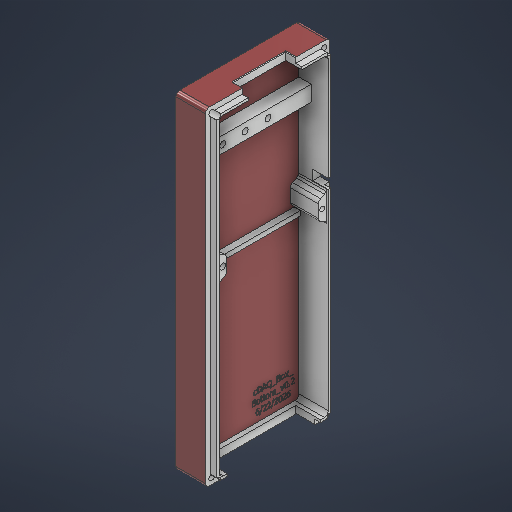
# Autodesk Inventor part: cDAQ_Box_Bottom_v0.2
Saved by Autodesk Inventor 2027 (Build 310192000, 192)
## iProperties
Created: 2026-05-08
Part Number: cDAQ_Box_Bottom_v0.2
Material: Generic
Document SubType Name: Modeling
Designer: giese
Density: 1 g/cm^3
Appearance: Default
Author: giese
Autodesk Inventor part; units mm, degrees
(part 1 of 2)
ref_plane "YZ Plane" through (0, 0, 0) normal (1, 0, 0) x (0, 1, 0)
ref_plane "XZ Plane" through (0, 0, 0) normal (0, 1, 0) x (-1, 0, 0)
ref_plane "XY Plane" through (0, 0, 0) normal (0, 0, 1) x (1, 0, 0)
sketch "Sketch1" plane through (0, 0, 0) normal (1, 0, 0) x (0, 1, 0)
  line L0 (37.5698, 53.1667) -> (-230.1462, 53.1667)
  line L1 (-230.1462, 53.1667) -> (-230.1462, -48.4333)
  line L2 (-230.1462, -48.4333) -> (37.5698, -48.4333)
  line L3 (37.5698, -48.4333) -> (37.5698, 53.1667)
  point P0 (0, 0)
  dimension "d0" = 101.6
  dimension "d1" = 267.716
  constraints: 8 end point, 2 parallel, 1 horizontal, 1 perpendicular
  measures "d0" distance of L2.end L0.start
  measures "d1" distance of L1.end L2.end
extrude "Extrusion1" add sketch "Sketch1" along normal blind 24.13
sketch "Sketch2" plane through (24.13, 0, 0) normal (1, 0, 0) x (0, 0, -1)
  line L0 (42.0833, 31.2198) -> (-46.8167, 31.2198)
  line L1 (-46.8167, 31.2198) -> (-46.8167, -223.7962)
  line L2 (-46.8167, -223.7962) -> (42.0833, -223.7962)
  line L3 (42.0833, -223.7962) -> (42.0833, 31.2198)
  line L4 (48.4333, 37.5698) -> (-53.1667, 37.5698) projected
  line L5 (-53.1667, 37.5698) -> (-53.1667, -230.1462) projected
  line L6 (-53.1667, -230.1462) -> (48.4333, -230.1462) projected
  point P0 (0, 0)
  dimension "d4" = 255.016
  dimension "d5" = 88.9
  dimension "d8" = 6.35
  dimension "d21" = 6.35
  dimension "d690" = 6.35
  constraints: 8 end point, 2 parallel, 1 horizontal, 1 perpendicular
  measures "d4" distance of L2.end L0.start
  measures "d5" distance of L0.start L0.end
  measures "d8" distance between parallel lines of L0 L4
  measures "d21" distance between parallel lines of L5 L1
  measures "d690" distance between parallel lines of L6 L2
extrude "Extrusion2" cut sketch "Sketch2" against normal blind 19.05
sketch "Sketch3" plane through (0, 0, 0) normal (-1, 0, 0) x (0, 0, 1)
  circle A0 centre (-6.6909, -3.0702) radius 2.4005
  circle A1 centre (11.8079, -3.0702) radius 2.4005
  circle A2 centre (30.3067, -3.0702) radius 2.4005
  line L0 (-48.4333, -230.1462) -> (-48.4333, 37.5698) projected
  line L1 (-48.4333, 37.5698) -> (53.1667, 37.5698) projected
  line L2 (53.1667, 37.5698) -> (53.1667, -230.1462) projected
  line L3 (46.8167, 31.2198) -> (-42.0833, 31.2198) projected
  point P0 (0, 0)
  point P1 (-0.896, -23.7433)
  point P2 (-45.1848, 27.0137)
  dimension "d9" = 18.4988
  dimension "d10" = 4.801
  dimension "d11" = 4.801
  dimension "d12" = 18.4988
  dimension "d13" = 36.9976
  dimension "d18" = 22.86
  dimension "d22" = 4.801
  dimension "d58" = 40.64
  constraints: 3 centre point
  measures "d9" distance of A0.centre A1.centre
  measures "d10" diameter of A1
  measures "d11" diameter of A2
  measures "d12" distance of A1.centre A2.centre
  measures "d13" distance of A0.centre A2.centre
  measures "d18" distance from line of L2 A2.centre
  measures "d22" diameter of A0
  measures "d58" distance from line of L1 A2.centre
extrude "Extrusion3" cut sketch "Sketch3" against normal blind 5.08
sketch "Sketch5" plane through (0, -230.1462, -48.4333) normal (0, 0, -1) x (-1, 0, 0)
  line L0 (-27.2034, 165.862) -> (-16.51, 165.862)
  line L1 (-16.51, 165.862) -> (-16.51, 173.862)
  line L2 (-16.51, 173.862) -> (-27.2034, 173.862)
  line L3 (-27.2034, 173.862) -> (-27.2034, 165.862)
  line L4 (0, 267.716) -> (-24.13, 267.716) projected
  line L5 (0, 0) -> (0, 267.716) projected
  line L6 (-24.13, 0) -> (-24.13, 267.716) projected
  point P0 (0, 230.1462)
  point P1 (-21.8567, 173.862)
  point P2 (-21.8567, 165.862)
  dimension "d28" = 10.6934
  dimension "d30" = 8
  dimension "d31" = 16.51
  dimension "d34" = 101.854
  dimension "d215" = 3.0734
  constraints: 8 end point, 2 midpoint, 2 parallel, 1 horizontal, 1 perpendicular
  measures "d28" distance between parallel lines of L1 L3
  measures "d30" distance of point (-21.857, 173.862) point (-21.857, 165.862)
  measures "d31" distance between parallel lines of L5 L1
  measures "d34" distance between parallel lines of L4 L0
  measures "d215" distance between parallel lines of L6 L3
extrude "Extrusion4" cut sketch "Sketch5" against normal blind 24.13
sketch "Sketch6" plane through (0, -230.1462, -48.4333) normal (0, -1, 0) x (1, 0, 0)
  line L0 (24.08, 55.136) -> (16.08, 55.136)
  line L1 (16.08, 45.136) -> (24.08, 45.136)
  line L2 (0, 101.6) -> (0, 0) projected
  line L3 (29.63, 53.1359) -> (29.63, 47.136)
  line L4 (24.08, 55.136) -> (29.63, 53.1359)
  line L5 (29.63, 47.136) -> (24.08, 45.136)
  line L6 (0, 0) -> (24.13, 0) projected
  line L7 (24.13, 95.25) -> (24.13, 6.35) projected
  line L8 (24.13, 41.9134) -> (24.13, 37.4697)
  line L9 (16.08, 55.136) -> (8.636, 55.136)
  line L10 (8.636, 55.136) -> (8.636, 45.136)
  line L11 (8.636, 45.136) -> (21.16, 45.136)
  point P0 (0, 48.4333)
  point P1 (20.08, 55.136)
  point P2 (20.08, 45.136)
  point P3 (16.08, 50.136)
  dimension "d39" = 6
  dimension "d48" = 55.136
  dimension "d221" = 0
  dimension "d223" = 2
  dimension "d224" = 2
  dimension "d225" = 5.5
  dimension "d227" = 5.55
  dimension "d672" = 8.636
  constraints: 18 end point, 2 horizontal, 2 midpoint, 2 parallel, 2 point on line, 1 perpendicular, 1 vertical
  measures "d39" distance of L3.start L3.end
  measures "d48" distance between parallel lines of L6 L0
  measures "d221" horizontal distance of L0.start L1.end
  measures "d223" vertical distance of L3.end L1.end
  measures "d224" vertical distance of L0.start L3.start
  measures "d225" distance between parallel lines of L3 L7
  measures "d227" distance from line of L1.end L3
  measures "d672" distance between parallel lines of L2 L10
extrude "Extrusion5" [suppressed]
sketch "Sketch7" plane through (0, 37.5698, 53.1667) normal (0, 1, 0) x (1, 0, 0)
  line L0 (32.512, 73.66) -> (16.002, 73.66)
  line L1 (16.002, 73.66) -> (16.002, 30.48)
  line L2 (16.002, 30.48) -> (32.512, 30.48)
  line L3 (32.512, 30.48) -> (32.512, 73.66)
  line L4 (0, 0) -> (24.13, 0) projected
  line L5 (0, 101.6) -> (0, 0) projected
  line L6 (24.13, 101.6) -> (24.13, 0) projected
  point P0 (0, 53.1667)
  point P1 (24.13, 73.66)
  point P2 (24.13, 30.48)
  dimension "d51" = 43.18
  dimension "d52" = 30.48
  dimension "d55" = 16.002
  dimension "d56" = 16.51
  dimension "d57" = 8.382
  constraints: 8 end point, 2 parallel, 1 horizontal, 1 perpendicular
  measures "d51" distance of L2.end L0.start
  measures "d52" distance between parallel lines of L4 L2
  measures "d55" distance between parallel lines of L5 L1
  measures "d56" distance between parallel lines of L3 L1
  measures "d57" distance between parallel lines of L6 L3
extrude "Extrusion6" cut sketch "Sketch7" against normal blind 7.62
fillet "Fillet1" radius 3.175 4 edges at (12.065, 37.5698, -48.4333) (12.065, 37.5698, 53.1667) (12.065, -230.1462, -48.4333) (12.065, -230.1462, 53.1667)
sketch "Sketch8" plane through (0, 0, 0) normal (-1, 0, 0) x (0, 0, 1)
  line L0 (-8.4625, -6.6008) -> (-4.9319, -6.6008)
  line L1 (-8.4625, 0.4604) -> (-4.9319, 0.4604)
  line L2 (-8.4625, -6.6008) -> (-10.5009, -3.0702)
  line L3 (-8.4625, 0.4604) -> (-10.5009, -3.0702)
  line L4 (-4.9319, -6.6008) -> (-2.8936, -3.0702)
  line L5 (-4.9319, 0.4604) -> (-2.8936, -3.0702)
  circle A0 centre (-6.6909, -3.0702) radius 2.4005 projected
  line L6 (10.0363, -6.6008) -> (13.5669, -6.6008)
  line L7 (10.0363, 0.4604) -> (13.5669, 0.4604)
  line L8 (10.0363, -6.6008) -> (7.9979, -3.0702)
  line L9 (10.0363, 0.4604) -> (7.9979, -3.0702)
  line L10 (13.5669, -6.6008) -> (15.6053, -3.0702)
  line L11 (13.5669, 0.4604) -> (15.6053, -3.0702)
  circle A1 centre (11.8079, -3.0702) radius 2.4005 projected
  line L12 (28.5351, -6.6008) -> (26.4967, -3.0702)
  line L13 (28.5351, 0.4604) -> (26.4967, -3.0702)
  line L14 (28.5351, -6.6008) -> (32.0657, -6.6008)
  line L15 (28.5351, 0.4604) -> (32.0657, 0.4604)
  line L16 (32.0657, -6.6008) -> (34.1041, -3.0702)
  line L17 (32.0657, 0.4604) -> (34.1041, -3.0702)
  circle A2 centre (30.3067, -3.0702) radius 2.4005 projected
  point P0 (-6.6972, -6.6008)
  point P1 (11.8016, -6.6008)
  point P2 (30.3004, -6.6008)
  point P3 (-10.5009, -3.0702)
  point P4 (-2.8936, -3.0702)
  point P5 (15.6053, -3.0702)
  point P6 (7.9979, -3.0702)
  point P7 (34.1041, -3.0702)
  point P8 (26.4967, -3.0702)
  dimension "d60" = 7.0612
  dimension "d61" = 120
  dimension "d62" = 120
  dimension "d63" = 120
  dimension "d64" = 120
  dimension "d65" = 3.5306
  dimension "d66" = 3.5306
  dimension "d67" = 3.5306
  dimension "d68" = 3.5306
  dimension "d69" = 3.5306
  dimension "d70" = 3.5306
  dimension "d71" = 0
  dimension "d72" = 7.6074
  dimension "d73" = 3.81
  dimension "d74" = 0
  dimension "d75" = 7.0612
  dimension "d76" = 120
  dimension "d77" = 120
  dimension "d78" = 120
  dimension "d79" = 120
  dimension "d80" = 3.5306
  dimension "d81" = 3.5306
  dimension "d82" = 3.5306
  dimension "d83" = 3.5306
  dimension "d84" = 3.5306
  dimension "d85" = 3.5306
  dimension "d86" = 0
  dimension "d87" = 7.6074
  dimension "d91" = 0
  dimension "d92" = 3.81
  dimension "d93" = 7.0612
  dimension "d94" = 120
  dimension "d95" = 120
  dimension "d96" = 120
  dimension "d97" = 120
  dimension "d98" = 3.5306
  dimension "d99" = 3.5306
  dimension "d100" = 3.5306
  dimension "d101" = 3.5306
  dimension "d102" = 3.5306
  dimension "d103" = 3.5306
  dimension "d104" = 0
  dimension "d105" = 7.6074
  dimension "d108" = 0
  dimension "d109" = 3.81
  constraints: 36 end point, 6 horizontal, 3 midpoint
  measures "d60" distance from line of point (-6.697, -6.601) L1
  measures "d61" angle of L0 L2
  measures "d62" angle of L1 L3
  measures "d63" angle of L4 L0
  measures "d64" angle of L5 L1
  measures "d65" distance of L0.start L0.end
  measures "d66" distance of L1.start L1.end
  measures "d67" vertical distance of L1.start L3.end
  measures "d68" vertical distance of L0.start L2.end
  measures "d69" vertical distance of L1.end L5.end
  measures "d70" vertical distance of L0.end L4.end
  measures "d71" horizontal distance of L0.start L1.start
  measures "d72" distance of L4.end L2.end
  measures "d73" distance of A0.centre L2.end
  measures "d74" vertical distance of A0.centre L4.end
  measures "d75" distance from line of point (11.802, -6.601) L7
  measures "d76" angle of L6 L8
  measures "d77" angle of L7 L9
  measures "d78" angle of L10 L6
  measures "d79" angle of L11 L7
  measures "d80" distance of L8.start L6.end
  measures "d81" distance of L9.start L7.end
  measures "d82" vertical distance of L9.start L9.end
  measures "d83" vertical distance of L8.start L8.end
  measures "d84" vertical distance of L7.end L11.end
  measures "d85" vertical distance of L6.end L10.end
  measures "d86" horizontal distance of L8.start L9.start
  measures "d87" distance of L10.end L8.end
  measures "d91" vertical distance of A1.centre L8.end
  measures "d92" distance of A1.centre L8.end
  measures "d93" distance from line of point (30.3, -6.601) L15
  measures "d94" angle of L14 L12
  measures "d95" angle of L15 L13
  measures "d96" angle of L16 L14
  measures "d97" angle of L17 L15
  measures "d98" distance of L12.start L16.start
  measures "d99" distance of L15.start L15.end
  measures "d100" vertical distance of L15.start L13.end
  measures "d101" vertical distance of L12.start L12.end
  measures "d102" vertical distance of L15.end L17.end
  measures "d103" vertical distance of L16.start L16.end
  measures "d104" horizontal distance of L12.start L15.start
  measures "d105" distance of L16.end L12.end
  measures "d108" vertical distance of A2.centre L12.end
  measures "d109" distance of A2.centre L12.end
extrude "Extrusion7" cut sketch "Sketch8" against normal blind 4 contours L2 L3 L1 L5 L4 L0 | A0 | L8 L9 L7 L11 L10 L6 | A1 | L12 L13 L15 L17 L16 L14 | A2
sketch "Sketch9" plane through (5.08, 0, 0) normal (1, 0, 0) x (0, 0, -1)
  arc A0 (24.8089, -180.8044) -> (19.3527, -180.8044) centre (22.0808, -178.3302) ccw
  line L0 (45.2583, 37.5698) -> (20.4933, 37.5698) projected
  line L1 (42.0833, 31.2198) -> (42.0833, -223.7962) projected
  arc A1 (20.1758, -185.9502) -> (23.9858, -185.9502) centre (22.0808, -185.9502) ccw
  line L2 (23.9858, -185.9502) -> (23.9858, -182.9374)
  line L3 (20.1758, -185.9502) -> (20.1758, -182.9374)
  arc A2 (24.8089, -180.8044) -> (23.9858, -182.9374) centre (27.1608, -182.9374) ccw
  arc A3 (20.1758, -182.9374) -> (19.3527, -180.8044) centre (17.0008, -182.9374) ccw
  arc A4 (-25.9911, -180.8044) -> (-31.4473, -180.8045) centre (-28.7192, -178.3302) ccw
  arc A5 (-30.6242, -185.9366) -> (-26.8142, -185.9502) centre (-28.7192, -185.9502) ccw
  line L4 (-26.8142, -185.9502) -> (-26.8142, -182.9374)
  line L5 (-30.6242, -185.9366) -> (-30.6242, -182.9374)
  arc A6 (-25.9911, -180.8044) -> (-26.8142, -182.9374) centre (-23.6392, -182.9374) ccw
  arc A7 (-30.6242, -182.9374) -> (-31.4473, -180.8045) centre (-33.7992, -182.9374) ccw
  line L6 (-22.6867, 37.5698) -> (-49.9917, 37.5698) projected
  line L7 (-46.8167, -223.7962) -> (-46.8167, 31.2198) projected
  point P0 (0, 0)
  point P1 (23.9858, -181.4823)
  point P2 (20.1758, -181.4823)
  point P3 (-26.8142, -181.4823)
  point P4 (-30.6242, -181.4823)
  dimension "d112" = 215.9
  dimension "d114" = 7.366
  dimension "d116" = 3.81
  dimension "d117" = 223.52
  dimension "d118" = 3.175
  dimension "d119" = 7.366
  dimension "d120" = 3.81
  dimension "d121" = 3.175
  dimension "d122" = 215.9
  dimension "d123" = 223.52
  dimension "d125" = 0
  dimension "d128" = 50.8
  dimension "d129" = 20.0025
  dimension "d130" = 0
  constraints: 20 point on circle, 8 centre point, 8 end point, 8 tangent, 4 point on line, 2 equal radius, 2 parallel, 2 vertical
  measures "d112" distance from line of L0 A0.centre
  measures "d114" diameter of A0
  measures "d116" diameter of A1
  measures "d117" distance from line of L0 A1.centre
  measures "d118" radius of A2
  measures "d119" diameter of A4
  measures "d120" diameter of A5
  measures "d121" radius of A6
  measures "d122" distance from line of A4.centre L6
  measures "d123" distance from line of L6 A5.centre
  measures "d125" horizontal distance of A5.centre A4.centre
  measures "d128" distance of A5.centre A1.centre
  measures "d129" distance from line of L1 A0.centre
  measures "d130" horizontal distance of A0.centre A1.centre
extrude "Extrusion8" [suppressed]
sketch "Sketch10" plane through (24.13, 0, 0) normal (1, 0, 0) x (0, 0, -1)
  line L0 (-46.8167, 31.2198) -> (42.0833, 31.2198) projected
  line L1 (-46.8167, 31.2198) -> (42.0833, 31.2198)
  line L2 (42.0833, 33.2264) -> (-46.8167, 33.2264)
  line L3 (-46.8167, 33.2264) -> (-48.8233, 33.2264)
  line L4 (-48.8233, 33.2264) -> (-48.8233, -225.8028)
  line L5 (-48.8233, -225.8028) -> (44.0899, -225.8028)
  line L6 (44.0899, -225.8028) -> (44.0899, 33.2264)
  line L7 (44.0899, 33.2264) -> (41.9392, 33.2264)
  line L8 (42.0833, 31.2198) -> (42.0833, -223.7962) projected
  line L9 (-46.8167, -223.7962) -> (-46.8167, 31.2198) projected
  line L10 (42.0833, -223.7962) -> (-46.8167, -223.7962) projected
  line L11 (45.2583, 37.5698) -> (20.4933, 37.5698) projected
  dimension "d202" = 2.0066
  dimension "d203" = 2.0066
  dimension "d204" = 2.0066
  dimension "d205" = 2.0066
  dimension "d208" = 4.3434
  constraints: 14 end point, 3 perpendicular, 3 point on line, 1 collinear, 1 horizontal
  measures "d202" distance between parallel lines of L0 L2
  measures "d203" distance between parallel lines of L6 L8
  measures "d204" distance between parallel lines of L4 L9
  measures "d205" distance between parallel lines of L5 L10
  measures "d208" distance between parallel lines of L11 L2
extrude "Extrusion9" add sketch "Sketch10" along normal blind 5
fillet "Fillet2" radius 3.175 8 edges at (17.105, 31.2198, -42.0833) (17.105, 31.2198, 46.8167) (17.105, -223.7962, 46.8167) (17.105, -223.7962, -42.0833) (26.63, 33.2264, -44.0899) (26.63, 33.2264, 48.8233) (26.63, -225.8028, -44.0899) (26.63, -225.8028, 48.8233)
sketch "Sketch13" plane through (29.13, 0, 0) normal (1, 0, 0) x (0, 0, -1)
  arc A0 (44.0833, 30.0448) -> (40.9083, 33.2198) centre (40.9083, 30.0448) ccw projected
  arc A1 (-45.6417, 33.2198) -> (-48.8167, 30.0448) centre (-45.6417, 30.0448) ccw projected
  arc A2 (40.9083, -212.0802) -> (44.0833, -208.9052) centre (40.9083, -208.9052) ccw projected
  arc A3 (-48.8167, -208.9052) -> (-45.6417, -212.0802) centre (-45.6417, -208.9052) ccw projected
  line L0 (-22.6867, 37.5698) -> (-49.9917, 37.5698) projected
  line L1 (-53.1667, 34.3948) -> (-53.1667, -226.9712) projected
  line L2 (-49.9917, -230.1462) -> (45.2583, -230.1462) projected
  arc A4 (-48.8167, -208.9052) -> (-45.6417, -212.0802) centre (-45.6417, -208.9052) ccw projected
  circle A5 centre (-48.0867, -225.0662) radius 2.4005
  circle A6 centre (43.3533, -225.0662) radius 2.4005
  line L3 (48.4333, -226.9712) -> (48.4333, 34.3948) projected
  circle A7 centre (43.3533, 32.4898) radius 2.4005
  line L4 (45.2583, 37.5698) -> (20.4933, 37.5698) projected
  circle A8 centre (-48.0867, 32.4898) radius 2.4005
  arc A9 (41.4904, -28.6131) -> (38.3154, -25.4381) centre (38.3154, -28.6131) ccw
  circle A10 centre (38.2733, -76.7302) radius 2.4005
  circle A11 centre (-43.0067, -76.7302) radius 2.4005
  point P0 (0, 0)
  point P1 (-47.8868, 32.2898)
  point P2 (-47.8868, -211.1503)
  point P3 (-47.8868, -211.1503)
  point P4 (45.8404, -24.2631)
  point P5 (42.6654, -21.0881)
  dimension "d178" = 5.08
  dimension "d179" = 5.08
  dimension "d180" = 4.801
  dimension "d181" = 5.08
  dimension "d182" = 5.08
  dimension "d183" = 4.801
  dimension "d184" = 4.801
  dimension "d185" = 5.08
  dimension "d186" = 5.08
  dimension "d187" = 4.801
  dimension "d188" = 5.08
  dimension "d189" = 5.08
  dimension "d326" = 4.801
  dimension "d327" = 10.16
  dimension "d328" = 114.3
  dimension "d329" = 4.801
  dimension "d330" = 10.16
  dimension "d331" = 114.3
  constraints: 7 centre point, 5 point on circle
  measures "d178" distance from line of L1 A5.centre
  measures "d179" distance from line of L2 A5.centre
  measures "d180" diameter of A5
  measures "d181" distance from line of L2 A6.centre
  measures "d182" distance from line of L3 A6.centre
  measures "d183" diameter of A6
  measures "d184" diameter of A7
  measures "d185" distance from line of L3 A7.centre
  measures "d186" distance from line of L4 A7.centre
  measures "d187" diameter of A8
  measures "d188" distance from line of L0 A8.centre
  measures "d189" distance from line of L1 A8.centre
  measures "d326" diameter of A10
  measures "d327" distance from line of L3 A10.centre
  measures "d328" distance from line of A10.centre L4
  measures "d329" diameter of A11
  measures "d330" distance from line of L1 A11.centre
  measures "d331" distance from line of L0 A11.centre
extrude "Extrusion11" cut sketch "Sketch13" against normal blind 25.4
sketch "Sketch14" plane through (5.08, 0, 0) normal (1, 0, 0) x (0, 0, -1)
  line L0 (11.5819, -199.2242) -> (30.7986, -199.2242) construction
  line L1 (30.7986, -199.2242) -> (30.7986, -197.2748) construction
  line L2 (30.7986, -197.2748) -> (11.5819, -197.2748) construction
  line L3 (11.5819, -197.2748) -> (11.5819, -199.2242) construction
  spline S0 degree 2 poles (6.6851, -203.9704) (6.3294, -203.9704) (5.7403, -203.7518) (5.5291, -203.5295) knots 0 0 0 1 2 2 2
  spline S1 degree 2 poles (5.5291, -203.5295) (5.3179, -203.3109) (5.0845, -202.6366) (5.0845, -202.1846) knots 0 0 0 1 2 2 2
  spline S2 degree 2 poles (5.0845, -202.1846) (5.0845, -201.7325) (5.3253, -201.073) (5.5291, -200.8507) knots 0 0 0 1 2 2 2
  spline S3 degree 2 poles (5.5291, -200.8507) (5.7329, -200.6247) (6.3368, -200.3839) (6.6851, -200.3839) knots 0 0 0 1 2 2 2
  spline S4 degree 2 poles (6.6851, -200.3839) (6.9667, -200.3839) (7.4928, -200.5432) (7.6966, -200.647) knots 0 0 0 1 2 2 2
  line L4 (7.6966, -200.647) -> (7.6966, -201.2953)
  line L5 (7.6966, -201.2953) -> (7.6632, -201.2953)
  spline S5 degree 2 poles (7.6632, -201.2953) (7.6002, -201.2435) (7.4076, -201.1101) (7.2705, -201.0397) knots 0 0 0 1 2 2 2
  spline S6 degree 2 poles (7.2705, -201.0397) (7.1482, -200.9804) (6.8222, -200.8878) (6.674, -200.8878) knots 0 0 0 1 2 2 2
  spline S7 degree 2 poles (6.674, -200.8878) (6.2257, -200.8878) (5.681, -201.5658) (5.681, -202.1846) knots 0 0 0 1 2 2 2
  spline S8 degree 2 poles (5.681, -202.1846) (5.681, -202.7885) (6.2071, -203.4665) (6.674, -203.4665) knots 0 0 0 1 2 2 2
  spline S9 degree 2 poles (6.674, -203.4665) (6.9556, -203.4665) (7.4668, -203.2331) (7.6632, -203.0515) knots 0 0 0 1 2 2 2
  line L6 (7.6632, -203.0515) -> (7.6966, -203.0515)
  line L7 (7.6966, -203.0515) -> (7.6966, -203.6999)
  spline S10 degree 2 poles (7.6966, -203.6999) (7.6113, -203.7407) (7.352, -203.8555) (7.2483, -203.8815) knots 0 0 0 1 2 2 2
  spline S11 degree 2 poles (7.2483, -203.8815) (7.1, -203.9259) (6.8666, -203.9704) (6.6851, -203.9704) knots 0 0 0 1 2 2 2
  spline S12 degree 2 poles (11.8721, -201.6103) (11.8721, -202.2364) (11.3645, -203.2442) (10.9385, -203.5258) knots 0 0 0 1 2 2 2
  spline S13 degree 2 poles (10.9385, -203.5258) (10.5902, -203.7444) (9.8751, -203.8926) (9.3194, -203.8926) knots 0 0 0 1 2 2 2
  line L8 (9.3194, -203.8926) -> (8.2671, -203.8926)
  line L9 (8.2671, -203.8926) -> (8.2671, -199.3206)
  line L10 (8.2671, -199.3206) -> (9.3082, -199.3206)
  spline S14 degree 2 poles (9.3082, -199.3206) (9.9529, -199.3206) (10.6865, -199.5132) (10.9459, -199.6837) knots 0 0 0 1 2 2 2
  spline S15 degree 2 poles (10.9459, -199.6837) (11.3868, -199.9764) (11.8721, -200.9434) (11.8721, -201.6103) knots 0 0 0 1 2 2 2
  spline S16 degree 2 poles (11.2386, -201.6029) (11.2386, -201.0767) (10.8903, -200.332) (10.5457, -200.1209) knots 0 0 0 1 2 2 2
  spline S17 degree 2 poles (10.5457, -200.1209) (10.3012, -199.9764) (9.7491, -199.8467) (9.3379, -199.8467) knots 0 0 0 1 2 2 2
  line L11 (9.3379, -199.8467) -> (8.8748, -199.8467)
  line L12 (8.8748, -199.8467) -> (8.8748, -203.3665)
  line L13 (8.8748, -203.3665) -> (9.3379, -203.3665)
  spline S18 degree 2 poles (9.3379, -203.3665) (9.7417, -203.3665) (10.3531, -203.2368) (10.6013, -203.0626) knots 0 0 0 1 2 2 2
  spline S19 degree 2 poles (10.6013, -203.0626) (10.9199, -202.8478) (11.2386, -202.1364) (11.2386, -201.6029) knots 0 0 0 1 2 2 2
  line L14 (12.0388, -203.8926) -> (13.5801, -199.3206)
  line L15 (13.5801, -199.3206) -> (14.3286, -199.3206)
  line L16 (14.3286, -199.3206) -> (15.8698, -203.8926)
  line L17 (15.8698, -203.8926) -> (15.2289, -203.8926)
  line L18 (15.2289, -203.8926) -> (14.8139, -202.6143)
  line L19 (14.8139, -202.6143) -> (13.0688, -202.6143)
  line L20 (13.0688, -202.6143) -> (12.6539, -203.8926)
  line L21 (12.6539, -203.8926) -> (12.0388, -203.8926)
  line L22 (14.6472, -202.0956) -> (13.9395, -199.943)
  line L23 (13.9395, -199.943) -> (13.2356, -202.0956)
  line L24 (13.2356, -202.0956) -> (14.6472, -202.0956)
  spline S20 degree 2 poles (20.101, -205.0115) (19.9343, -205.0522) (19.5712, -205.0967) (19.3896, -205.0967) knots 0 0 0 1 2 2 2
  spline S21 degree 2 poles (19.3896, -205.0967) (18.8746, -205.0967) (18.2336, -204.5224) (18.204, -203.9889) knots 0 0 0 1 2 2 2
  spline S22 degree 2 poles (18.204, -203.9889) (18.1633, -203.9889) (18.0929, -203.9889) (18.0632, -203.9889) knots 0 0 0 1 2 2 2
  spline S23 degree 2 poles (18.0632, -203.9889) (17.6001, -203.9889) (16.8554, -203.674) (16.5886, -203.3665) knots 0 0 0 1 2 2 2
  spline S24 degree 2 poles (16.5886, -203.3665) (16.3256, -203.0626) (16.044, -202.1734) (16.044, -201.6103) knots 0 0 0 1 2 2 2
  spline S25 degree 2 poles (16.044, -201.6103) (16.044, -201.0323) (16.3293, -200.1579) (16.5923, -199.8467) knots 0 0 0 1 2 2 2
  spline S26 degree 2 poles (16.5923, -199.8467) (16.8591, -199.5392) (17.6038, -199.2242) (18.0632, -199.2242) knots 0 0 0 1 2 2 2
  spline S27 degree 2 poles (18.0632, -199.2242) (18.53, -199.2242) (19.2785, -199.5503) (19.5378, -199.8467) knots 0 0 0 1 2 2 2
  spline S28 degree 2 poles (19.5378, -199.8467) (19.7972, -200.1468) (20.0862, -201.0397) (20.0862, -201.6103) knots 0 0 0 1 2 2 2
  spline S29 degree 2 poles (20.0862, -201.6103) (20.0862, -202.4995) (19.3933, -203.6554) (18.7894, -203.8592) knots 0 0 0 1 2 2 2
  spline S30 degree 2 poles (18.7894, -203.8592) (18.8042, -204.0297) (18.8931, -204.3038) (18.9635, -204.3816) knots 0 0 0 1 2 2 2
  spline S31 degree 2 poles (18.9635, -204.3816) (19.0488, -204.478) (19.2822, -204.5669) (19.4897, -204.5669) knots 0 0 0 1 2 2 2
  spline S32 degree 2 poles (19.4897, -204.5669) (19.6119, -204.5669) (19.9454, -204.4891) (20.0195, -204.4594) knots 0 0 0 1 2 2 2
  line L25 (20.0195, -204.4594) -> (20.101, -204.4594)
  line L26 (20.101, -204.4594) -> (20.101, -205.0115)
  spline S33 degree 2 poles (19.4526, -201.6103) (19.4526, -201.1546) (19.2562, -200.4543) (19.0784, -200.2246) knots 0 0 0 1 2 2 2
  spline S34 degree 2 poles (19.0784, -200.2246) (18.8968, -199.9875) (18.3856, -199.7504) (18.0669, -199.7504) knots 0 0 0 1 2 2 2
  spline S35 degree 2 poles (18.0669, -199.7504) (17.7372, -199.7504) (17.2407, -199.9801) (17.0517, -200.2246) knots 0 0 0 1 2 2 2
  spline S36 degree 2 poles (17.0517, -200.2246) (16.8702, -200.458) (16.6775, -201.1657) (16.6775, -201.6103) knots 0 0 0 1 2 2 2
  spline S37 degree 2 poles (16.6775, -201.6103) (16.6775, -202.5106) (17.4334, -203.4702) (18.0669, -203.4702) knots 0 0 0 1 2 2 2
  spline S38 degree 2 poles (18.0669, -203.4702) (18.7005, -203.4702) (19.4526, -202.5106) (19.4526, -201.6103) knots 0 0 0 1 2 2 2
  line L27 (23.769, -204.8114) -> (20.2418, -204.8114)
  line L28 (20.2418, -204.8114) -> (20.2418, -204.415)
  line L29 (20.2418, -204.415) -> (23.769, -204.415)
  line L30 (23.769, -204.415) -> (23.769, -204.8114)
  spline S39 degree 2 poles (27.285, -202.4884) (27.285, -202.8292) (27.0257, -203.3516) (26.8108, -203.5221) knots 0 0 0 1 2 2 2
  spline S40 degree 2 poles (26.8108, -203.5221) (26.5514, -203.7221) (25.9623, -203.8926) (25.4955, -203.8926) knots 0 0 0 1 2 2 2
  line L31 (25.4955, -203.8926) -> (24.1839, -203.8926)
  line L32 (24.1839, -203.8926) -> (24.1839, -199.3206)
  line L33 (24.1839, -199.3206) -> (25.3955, -199.3206)
  spline S41 degree 2 poles (25.3955, -199.3206) (25.8845, -199.3206) (26.3736, -199.3836) (26.5959, -199.5058) knots 0 0 0 1 2 2 2
  spline S42 degree 2 poles (26.5959, -199.5058) (26.8441, -199.6355) (27.0701, -200.0616) (27.0701, -200.3506) knots 0 0 0 1 2 2 2
  spline S43 degree 2 poles (27.0701, -200.3506) (27.0701, -200.6729) (26.7293, -201.1842) (26.4292, -201.3287) knots 0 0 0 1 2 2 2
  line L34 (26.4292, -201.3287) -> (26.4292, -201.3509)
  spline S44 degree 2 poles (26.4292, -201.3509) (26.8367, -201.4621) (27.285, -202.0512) (27.285, -202.4884) knots 0 0 0 1 2 2 2
  spline S45 degree 2 poles (26.6515, -202.5143) (26.6515, -202.2549) (26.5033, -201.9215) (26.281, -201.8029) knots 0 0 0 1 2 2 2
  spline S46 degree 2 poles (26.281, -201.8029) (26.1365, -201.7288) (25.7956, -201.6844) (25.4807, -201.6844) knots 0 0 0 1 2 2 2
  line L35 (25.4807, -201.6844) -> (24.7915, -201.6844)
  line L36 (24.7915, -201.6844) -> (24.7915, -203.3739)
  line L37 (24.7915, -203.3739) -> (25.2843, -203.3739)
  spline S47 degree 2 poles (25.2843, -203.3739) (25.6845, -203.3739) (26.1439, -203.2998) (26.3217, -203.1812) knots 0 0 0 1 2 2 2
  spline S48 degree 2 poles (26.3217, -203.1812) (26.4921, -203.0589) (26.6515, -202.7551) (26.6515, -202.5143) knots 0 0 0 1 2 2 2
  spline S49 degree 2 poles (26.4366, -200.4358) (26.4366, -200.2728) (26.3254, -200.0282) (26.2032, -199.9578) knots 0 0 0 1 2 2 2
  spline S50 degree 2 poles (26.2032, -199.9578) (26.055, -199.8763) (25.6956, -199.8393) (25.3732, -199.8393) knots 0 0 0 1 2 2 2
  line L38 (25.3732, -199.8393) -> (24.7915, -199.8393)
  line L39 (24.7915, -199.8393) -> (24.7915, -201.1768)
  line L40 (24.7915, -201.1768) -> (25.4807, -201.1768)
  spline S51 degree 2 poles (25.4807, -201.1768) (25.766, -201.1768) (26.0364, -201.1175) (26.1809, -201.0249) knots 0 0 0 1 2 2 2
  spline S52 degree 2 poles (26.1809, -201.0249) (26.3217, -200.936) (26.4366, -200.6507) (26.4366, -200.4358) knots 0 0 0 1 2 2 2
  spline S53 degree 2 poles (30.664, -202.1771) (30.664, -203.0441) (29.8304, -203.9889) (29.1338, -203.9889) knots 0 0 0 1 2 2 2
  spline S54 degree 2 poles (29.1338, -203.9889) (28.4188, -203.9889) (27.5999, -203.0145) (27.5999, -202.1771) knots 0 0 0 1 2 2 2
  spline S55 degree 2 poles (27.5999, -202.1771) (27.5999, -201.3176) (28.4447, -200.3654) (29.1338, -200.3654) knots 0 0 0 1 2 2 2
  spline S56 degree 2 poles (29.1338, -200.3654) (29.8304, -200.3654) (30.664, -201.3139) (30.664, -202.1771) knots 0 0 0 1 2 2 2
  spline S57 degree 2 poles (30.0675, -202.1771) (30.0675, -201.5102) (29.5821, -200.8619) (29.1338, -200.8619) knots 0 0 0 1 2 2 2
  spline S58 degree 2 poles (29.1338, -200.8619) (28.6855, -200.8619) (28.1965, -201.5102) (28.1965, -202.1771) knots 0 0 0 1 2 2 2
  spline S59 degree 2 poles (28.1965, -202.1771) (28.1965, -202.8255) (28.6855, -203.4924) (29.1338, -203.4924) knots 0 0 0 1 2 2 2
  spline S60 degree 2 poles (29.1338, -203.4924) (29.5784, -203.4924) (30.0675, -202.8366) (30.0675, -202.1771) knots 0 0 0 1 2 2 2
  line L41 (33.9207, -203.8926) -> (33.2131, -203.8926)
  line L42 (33.2131, -203.8926) -> (32.3794, -202.6032)
  line L43 (32.3794, -202.6032) -> (31.5236, -203.8926)
  line L44 (31.5236, -203.8926) -> (30.8678, -203.8926)
  line L45 (30.8678, -203.8926) -> (32.0571, -202.192)
  line L46 (32.0571, -202.192) -> (30.8789, -200.4617)
  line L47 (30.8789, -200.4617) -> (31.5866, -200.4617)
  line L48 (31.5866, -200.4617) -> (32.4165, -201.7399)
  line L49 (32.4165, -201.7399) -> (33.2649, -200.4617)
  line L50 (33.2649, -200.4617) -> (33.9207, -200.4617)
  line L51 (33.9207, -200.4617) -> (32.7388, -202.1549)
  line L52 (32.7388, -202.1549) -> (33.9207, -203.8926)
  line L53 (37.4294, -204.8114) -> (33.9022, -204.8114)
  line L54 (33.9022, -204.8114) -> (33.9022, -204.415)
  line L55 (33.9022, -204.415) -> (37.4294, -204.415)
  line L56 (37.4294, -204.415) -> (37.4294, -204.8114)
  spline S61 degree 2 poles (7.0815, -210.016) (7.0815, -210.3569) (6.8222, -210.8793) (6.6073, -211.0497) knots 0 0 0 1 2 2 2
  spline S62 degree 2 poles (6.6073, -211.0497) (6.3479, -211.2498) (5.7588, -211.4202) (5.292, -211.4202) knots 0 0 0 1 2 2 2
  line L57 (5.292, -211.4202) -> (3.9804, -211.4202)
  line L58 (3.9804, -211.4202) -> (3.9804, -206.8482)
  line L59 (3.9804, -206.8482) -> (5.192, -206.8482)
  spline S63 degree 2 poles (5.192, -206.8482) (5.681, -206.8482) (6.1701, -206.9112) (6.3924, -207.0335) knots 0 0 0 1 2 2 2
  spline S64 degree 2 poles (6.3924, -207.0335) (6.6406, -207.1632) (6.8666, -207.5892) (6.8666, -207.8782) knots 0 0 0 1 2 2 2
  spline S65 degree 2 poles (6.8666, -207.8782) (6.8666, -208.2006) (6.5258, -208.7119) (6.2257, -208.8564) knots 0 0 0 1 2 2 2
  line L60 (6.2257, -208.8564) -> (6.2257, -208.8786)
  spline S66 degree 2 poles (6.2257, -208.8786) (6.6332, -208.9897) (7.0815, -209.5788) (7.0815, -210.016) knots 0 0 0 1 2 2 2
  spline S67 degree 2 poles (6.448, -210.042) (6.448, -209.7826) (6.2998, -209.4492) (6.0775, -209.3306) knots 0 0 0 1 2 2 2
  spline S68 degree 2 poles (6.0775, -209.3306) (5.933, -209.2565) (5.5921, -209.2121) (5.2772, -209.2121) knots 0 0 0 1 2 2 2
  line L61 (5.2772, -209.2121) -> (4.588, -209.2121)
  line L62 (4.588, -209.2121) -> (4.588, -210.9015)
  line L63 (4.588, -210.9015) -> (5.0808, -210.9015)
  spline S69 degree 2 poles (5.0808, -210.9015) (5.481, -210.9015) (5.9404, -210.8274) (6.1182, -210.7089) knots 0 0 0 1 2 2 2
  spline S70 degree 2 poles (6.1182, -210.7089) (6.2886, -210.5866) (6.448, -210.2828) (6.448, -210.042) knots 0 0 0 1 2 2 2
  spline S71 degree 2 poles (6.2331, -207.9635) (6.2331, -207.8004) (6.1219, -207.5559) (5.9997, -207.4855) knots 0 0 0 1 2 2 2
  spline S72 degree 2 poles (5.9997, -207.4855) (5.8515, -207.404) (5.4921, -207.3669) (5.1697, -207.3669) knots 0 0 0 1 2 2 2
  line L64 (5.1697, -207.3669) -> (4.588, -207.3669)
  line L65 (4.588, -207.3669) -> (4.588, -208.7045)
  line L66 (4.588, -208.7045) -> (5.2772, -208.7045)
  spline S73 degree 2 poles (5.2772, -208.7045) (5.5625, -208.7045) (5.8329, -208.6452) (5.9774, -208.5526) knots 0 0 0 1 2 2 2
  spline S74 degree 2 poles (5.9774, -208.5526) (6.1182, -208.4636) (6.2331, -208.1783) (6.2331, -207.9635) knots 0 0 0 1 2 2 2
  spline S75 degree 2 poles (10.4605, -209.7048) (10.4605, -210.5718) (9.6269, -211.5166) (8.9303, -211.5166) knots 0 0 0 1 2 2 2
  spline S76 degree 2 poles (8.9303, -211.5166) (8.2153, -211.5166) (7.3965, -210.5422) (7.3965, -209.7048) knots 0 0 0 1 2 2 2
  spline S77 degree 2 poles (7.3965, -209.7048) (7.3965, -208.8453) (8.2412, -207.8931) (8.9303, -207.8931) knots 0 0 0 1 2 2 2
  spline S78 degree 2 poles (8.9303, -207.8931) (9.6269, -207.8931) (10.4605, -208.8415) (10.4605, -209.7048) knots 0 0 0 1 2 2 2
  spline S79 degree 2 poles (9.864, -209.7048) (9.864, -209.0379) (9.3786, -208.3895) (8.9303, -208.3895) knots 0 0 0 1 2 2 2
  spline S80 degree 2 poles (8.9303, -208.3895) (8.482, -208.3895) (7.993, -209.0379) (7.993, -209.7048) knots 0 0 0 1 2 2 2
  spline S81 degree 2 poles (7.993, -209.7048) (7.993, -210.3532) (8.482, -211.0201) (8.9303, -211.0201) knots 0 0 0 1 2 2 2
  spline S82 degree 2 poles (8.9303, -211.0201) (9.3749, -211.0201) (9.864, -210.3643) (9.864, -209.7048) knots 0 0 0 1 2 2 2
  spline S83 degree 2 poles (12.0907, -211.4869) (11.6202, -211.4869) (11.0904, -210.9497) (11.0904, -210.368) knots 0 0 0 1 2 2 2
  line L67 (11.0904, -210.368) -> (11.0904, -208.4673)
  line L68 (11.0904, -208.4673) -> (10.7013, -208.4673)
  line L69 (10.7013, -208.4673) -> (10.7013, -207.9894)
  line L70 (10.7013, -207.9894) -> (11.0904, -207.9894)
  line L71 (11.0904, -207.9894) -> (11.0904, -207.0039)
  line L72 (11.0904, -207.0039) -> (11.6683, -207.0039)
  line L73 (11.6683, -207.0039) -> (11.6683, -207.9894)
  line L74 (11.6683, -207.9894) -> (12.7317, -207.9894)
  line L75 (12.7317, -207.9894) -> (12.7317, -208.4673)
  line L76 (12.7317, -208.4673) -> (11.6683, -208.4673)
  line L77 (11.6683, -208.4673) -> (11.6683, -210.1013)
  spline S84 degree 2 poles (11.6683, -210.1013) (11.6683, -210.3606) (11.6869, -210.6459) (11.7499, -210.7682) knots 0 0 0 1 2 2 2
  spline S85 degree 2 poles (11.7499, -210.7682) (11.8017, -210.8756) (12.0351, -210.9831) (12.2352, -210.9831) knots 0 0 0 1 2 2 2
  spline S86 degree 2 poles (12.2352, -210.9831) (12.376, -210.9831) (12.6391, -210.8978) (12.6983, -210.8719) knots 0 0 0 1 2 2 2
  line L78 (12.6983, -210.8719) -> (12.7317, -210.8719)
  line L79 (12.7317, -210.8719) -> (12.7317, -211.3906)
  spline S87 degree 2 poles (12.7317, -211.3906) (12.5687, -211.4351) (12.2352, -211.4869) (12.0907, -211.4869) knots 0 0 0 1 2 2 2
  spline S88 degree 2 poles (14.1952, -211.4869) (13.7246, -211.4869) (13.1948, -210.9497) (13.1948, -210.368) knots 0 0 0 1 2 2 2
  line L80 (13.1948, -210.368) -> (13.1948, -208.4673)
  line L81 (13.1948, -208.4673) -> (12.8058, -208.4673)
  line L82 (12.8058, -208.4673) -> (12.8058, -207.9894)
  line L83 (12.8058, -207.9894) -> (13.1948, -207.9894)
  line L84 (13.1948, -207.9894) -> (13.1948, -207.0039)
  line L85 (13.1948, -207.0039) -> (13.7728, -207.0039)
  line L86 (13.7728, -207.0039) -> (13.7728, -207.9894)
  line L87 (13.7728, -207.9894) -> (14.8361, -207.9894)
  line L88 (14.8361, -207.9894) -> (14.8361, -208.4673)
  line L89 (14.8361, -208.4673) -> (13.7728, -208.4673)
  line L90 (13.7728, -208.4673) -> (13.7728, -210.1013)
  spline S89 degree 2 poles (13.7728, -210.1013) (13.7728, -210.3606) (13.7913, -210.6459) (13.8543, -210.7682) knots 0 0 0 1 2 2 2
  spline S90 degree 2 poles (13.8543, -210.7682) (13.9062, -210.8756) (14.1396, -210.9831) (14.3397, -210.9831) knots 0 0 0 1 2 2 2
  spline S91 degree 2 poles (14.3397, -210.9831) (14.4805, -210.9831) (14.7435, -210.8978) (14.8028, -210.8719) knots 0 0 0 1 2 2 2
  line L91 (14.8028, -210.8719) -> (14.8361, -210.8719)
  line L92 (14.8361, -210.8719) -> (14.8361, -211.3906)
  spline S92 degree 2 poles (14.8361, -211.3906) (14.6731, -211.4351) (14.3397, -211.4869) (14.1952, -211.4869) knots 0 0 0 1 2 2 2
  spline S93 degree 2 poles (18.0817, -209.7048) (18.0817, -210.5718) (17.2481, -211.5166) (16.5516, -211.5166) knots 0 0 0 1 2 2 2
  spline S94 degree 2 poles (16.5516, -211.5166) (15.8365, -211.5166) (15.0177, -210.5422) (15.0177, -209.7048) knots 0 0 0 1 2 2 2
  spline S95 degree 2 poles (15.0177, -209.7048) (15.0177, -208.8453) (15.8624, -207.8931) (16.5516, -207.8931) knots 0 0 0 1 2 2 2
  spline S96 degree 2 poles (16.5516, -207.8931) (17.2481, -207.8931) (18.0817, -208.8415) (18.0817, -209.7048) knots 0 0 0 1 2 2 2
  spline S97 degree 2 poles (17.4852, -209.7048) (17.4852, -209.0379) (16.9999, -208.3895) (16.5516, -208.3895) knots 0 0 0 1 2 2 2
  spline S98 degree 2 poles (16.5516, -208.3895) (16.1033, -208.3895) (15.6142, -209.0379) (15.6142, -209.7048) knots 0 0 0 1 2 2 2
  spline S99 degree 2 poles (15.6142, -209.7048) (15.6142, -210.3532) (16.1033, -211.0201) (16.5516, -211.0201) knots 0 0 0 1 2 2 2
  spline S100 degree 2 poles (16.5516, -211.0201) (16.9962, -211.0201) (17.4852, -210.3643) (17.4852, -209.7048) knots 0 0 0 1 2 2 2
  line L93 (22.5648, -211.4202) -> (22.5648, -209.4344)
  spline S101 degree 2 poles (22.5648, -209.4344) (22.5648, -209.1972) (22.5278, -208.7934) (22.4685, -208.6822) knots 0 0 0 1 2 2 2
  spline S102 degree 2 poles (22.4685, -208.6822) (22.4092, -208.56) (22.1832, -208.4414) (21.9868, -208.4414) knots 0 0 0 1 2 2 2
  spline S103 degree 2 poles (21.9868, -208.4414) (21.809, -208.4414) (21.4014, -208.66) (21.1866, -208.8675) knots 0 0 0 1 2 2 2
  spline S104 degree 2 poles (21.1866, -208.8675) (21.1903, -208.9194) (21.1977, -209.0638) (21.1977, -209.1602) knots 0 0 0 1 2 2 2
  line L94 (21.1977, -209.1602) -> (21.1977, -211.4202)
  line L95 (21.1977, -211.4202) -> (20.6197, -211.4202)
  line L96 (20.6197, -211.4202) -> (20.6197, -209.4344)
  spline S105 degree 2 poles (20.6197, -209.4344) (20.6197, -209.1972) (20.5826, -208.7934) (20.5234, -208.6822) knots 0 0 0 1 2 2 2
  spline S106 degree 2 poles (20.5234, -208.6822) (20.4641, -208.56) (20.2381, -208.4414) (20.0417, -208.4414) knots 0 0 0 1 2 2 2
  spline S107 degree 2 poles (20.0417, -208.4414) (19.8564, -208.4414) (19.4452, -208.6748) (19.2525, -208.8564) knots 0 0 0 1 2 2 2
  line L97 (19.2525, -208.8564) -> (19.2525, -211.4202)
  line L98 (19.2525, -211.4202) -> (18.6745, -211.4202)
  line L99 (18.6745, -211.4202) -> (18.6745, -207.9894)
  line L100 (18.6745, -207.9894) -> (19.2525, -207.9894)
  line L101 (19.2525, -207.9894) -> (19.2525, -208.3673)
  spline S108 degree 2 poles (19.2525, -208.3673) (19.4785, -208.1413) (19.9231, -207.8931) (20.1899, -207.8931) knots 0 0 0 1 2 2 2
  spline S109 degree 2 poles (20.1899, -207.8931) (20.4937, -207.8931) (20.9643, -208.1709) (21.0865, -208.4859) knots 0 0 0 1 2 2 2
  spline S110 degree 2 poles (21.0865, -208.4859) (21.3496, -208.1932) (21.846, -207.8931) (22.135, -207.8931) knots 0 0 0 1 2 2 2
  spline S111 degree 2 poles (22.135, -207.8931) (22.3573, -207.8931) (22.7204, -208.0301) (22.8538, -208.1858) knots 0 0 0 1 2 2 2
  spline S112 degree 2 poles (22.8538, -208.1858) (22.9909, -208.3414) (23.1428, -208.8082) (23.1428, -209.1602) knots 0 0 0 1 2 2 2
  line L102 (23.1428, -209.1602) -> (23.1428, -211.4202)
  line L103 (23.1428, -211.4202) -> (22.5648, -211.4202)
  line L104 (27.0146, -212.3391) -> (23.4874, -212.3391)
  line L105 (23.4874, -212.3391) -> (23.4874, -211.9427)
  line L106 (23.4874, -211.9427) -> (27.0146, -211.9427)
  line L107 (27.0146, -211.9427) -> (27.0146, -212.3391)
  line L108 (30.0786, -207.9894) -> (28.7856, -211.4202)
  line L109 (28.7856, -211.4202) -> (28.2669, -211.4202)
  line L110 (28.2669, -211.4202) -> (26.9849, -207.9894)
  line L111 (26.9849, -207.9894) -> (27.6111, -207.9894)
  line L112 (27.6111, -207.9894) -> (28.5484, -210.6311)
  line L113 (28.5484, -210.6311) -> (29.4784, -207.9894)
  line L114 (29.4784, -207.9894) -> (30.0786, -207.9894)
  spline S113 degree 2 poles (33.276, -209.1342) (33.276, -210.3643) (32.561, -211.5166) (31.8163, -211.5166) knots 0 0 0 1 2 2 2
  spline S114 degree 2 poles (31.8163, -211.5166) (31.0604, -211.5166) (30.3528, -210.3421) (30.3528, -209.1379) knots 0 0 0 1 2 2 2
  spline S115 degree 2 poles (30.3528, -209.1379) (30.3528, -207.9005) (31.0679, -206.7556) (31.8163, -206.7556) knots 0 0 0 1 2 2 2
  spline S116 degree 2 poles (31.8163, -206.7556) (32.5684, -206.7556) (33.276, -207.9412) (33.276, -209.1342) knots 0 0 0 1 2 2 2
  spline S117 degree 2 poles (32.4906, -210.5273) (32.5795, -210.3013) (32.6536, -209.6048) (32.6536, -209.1342) knots 0 0 0 1 2 2 2
  spline S118 degree 2 poles (32.6536, -209.1342) (32.6536, -208.6637) (32.5795, -207.9709) (32.4869, -207.7375) knots 0 0 0 1 2 2 2
  spline S119 degree 2 poles (32.4869, -207.7375) (32.3943, -207.504) (32.0719, -207.2632) (31.8163, -207.2632) knots 0 0 0 1 2 2 2
  spline S120 degree 2 poles (31.8163, -207.2632) (31.5606, -207.2632) (31.2309, -207.504) (31.1345, -207.7449) knots 0 0 0 1 2 2 2
  spline S121 degree 2 poles (31.1345, -207.7449) (31.0419, -207.9783) (30.9752, -208.6896) (30.9752, -209.1379) knots 0 0 0 1 2 2 2
  spline S122 degree 2 poles (30.9752, -209.1379) (30.9752, -209.6196) (31.0345, -210.2643) (31.1308, -210.5162) knots 0 0 0 1 2 2 2
  spline S123 degree 2 poles (31.1308, -210.5162) (31.2198, -210.7533) (31.5495, -211.009) (31.8163, -211.009) knots 0 0 0 1 2 2 2
  spline S124 degree 2 poles (31.8163, -211.009) (32.0682, -211.009) (32.398, -210.7682) (32.4906, -210.5273) knots 0 0 0 1 2 2 2
  line L115 (34.8433, -211.4202) -> (34.1097, -211.4202)
  line L116 (34.1097, -211.4202) -> (34.1097, -210.5459)
  line L117 (34.1097, -210.5459) -> (34.8433, -210.5459)
  line L118 (34.8433, -210.5459) -> (34.8433, -211.4202)
  line L119 (38.5853, -211.4202) -> (35.7658, -211.4202)
  line L120 (35.7658, -211.4202) -> (35.7658, -210.7719)
  spline S125 degree 2 poles (35.7658, -210.7719) (36.0696, -210.4866) (36.6106, -209.9568) (36.8699, -209.6715) knots 0 0 0 1 2 2 2
  spline S126 degree 2 poles (36.8699, -209.6715) (37.3923, -209.0972) (37.7739, -208.4081) (37.7739, -208.0413) knots 0 0 0 1 2 2 2
  spline S127 degree 2 poles (37.7739, -208.0413) (37.7739, -207.8486) (37.6554, -207.5596) (37.5479, -207.467) knots 0 0 0 1 2 2 2
  spline S128 degree 2 poles (37.5479, -207.467) (37.4405, -207.3744) (37.1589, -207.2817) (36.9885, -207.2817) knots 0 0 0 1 2 2 2
  spline S129 degree 2 poles (36.9885, -207.2817) (36.8255, -207.2817) (36.492, -207.3632) (36.3401, -207.4262) knots 0 0 0 1 2 2 2
  spline S130 degree 2 poles (36.3401, -207.4262) (36.2104, -207.4781) (35.9696, -207.6263) (35.8955, -207.6782) knots 0 0 0 1 2 2 2
  line L121 (35.8955, -207.6782) -> (35.8622, -207.6782)
  line L122 (35.8622, -207.6782) -> (35.8622, -207.0261)
  spline S131 degree 2 poles (35.8622, -207.0261) (36.0511, -206.9335) (36.7291, -206.7519) (37.0329, -206.7519) knots 0 0 0 1 2 2 2
  spline S132 degree 2 poles (37.0329, -206.7519) (37.6739, -206.7519) (38.3964, -207.4299) (38.3964, -208.0079) knots 0 0 0 1 2 2 2
  spline S133 degree 2 poles (38.3964, -208.0079) (38.3964, -208.2784) (38.2704, -208.7304) (38.1593, -208.9231) knots 0 0 0 1 2 2 2
  spline S134 degree 2 poles (38.1593, -208.9231) (38.0481, -209.1231) (37.7258, -209.5159) (37.5479, -209.7048) knots 0 0 0 1 2 2 2
  spline S135 degree 2 poles (37.5479, -209.7048) (37.2589, -210.0197) (36.5513, -210.6941) (36.3401, -210.8904) knots 0 0 0 1 2 2 2
  line L123 (36.3401, -210.8904) -> (38.5853, -210.8904)
  line L124 (38.5853, -210.8904) -> (38.5853, -211.4202)
  spline S136 degree 2 poles (10.0011, -217.4659) (10.0011, -217.8179) (9.7677, -218.4144) (9.5713, -218.6145) knots 0 0 0 1 2 2 2
  spline S137 degree 2 poles (9.5713, -218.6145) (9.3675, -218.8257) (8.8562, -219.0443) (8.5487, -219.0443) knots 0 0 0 1 2 2 2
  spline S138 degree 2 poles (8.5487, -219.0443) (8.2412, -219.0443) (7.7336, -218.8368) (7.5409, -218.6293) knots 0 0 0 1 2 2 2
  spline S139 degree 2 poles (7.5409, -218.6293) (7.3038, -218.3811) (7.0371, -217.5474) (7.0371, -216.9398) knots 0 0 0 1 2 2 2
  spline S140 degree 2 poles (7.0371, -216.9398) (7.0371, -216.3433) (7.2816, -215.3837) (7.5372, -215.028) knots 0 0 0 1 2 2 2
  spline S141 degree 2 poles (7.5372, -215.028) (7.7855, -214.6797) (8.5709, -214.2907) (9.0859, -214.2907) knots 0 0 0 1 2 2 2
  spline S142 degree 2 poles (9.0859, -214.2907) (9.2378, -214.2907) (9.5046, -214.3203) (9.6046, -214.3537) knots 0 0 0 1 2 2 2
  line L125 (9.6046, -214.3537) -> (9.6046, -214.9428)
  line L126 (9.6046, -214.9428) -> (9.5787, -214.9428)
  spline S143 degree 2 poles (9.5787, -214.9428) (9.4935, -214.8983) (9.1823, -214.8205) (9.0044, -214.8205) knots 0 0 0 1 2 2 2
  spline S144 degree 2 poles (9.0044, -214.8205) (8.4339, -214.8205) (7.7336, -215.5912) (7.6669, -216.347) knots 0 0 0 1 2 2 2
  spline S145 degree 2 poles (7.6669, -216.347) (7.8855, -216.1951) (8.3449, -216.0284) (8.6191, -216.0284) knots 0 0 0 1 2 2 2
  spline S146 degree 2 poles (8.6191, -216.0284) (8.8859, -216.0284) (9.286, -216.1358) (9.5046, -216.2988) knots 0 0 0 1 2 2 2
  spline S147 degree 2 poles (9.5046, -216.2988) (9.7566, -216.4878) (10.0011, -217.0732) (10.0011, -217.4659) knots 0 0 0 1 2 2 2
  spline S148 degree 2 poles (9.3786, -217.4918) (9.3786, -217.2103) (9.2304, -216.8286) (9.0674, -216.6953) knots 0 0 0 1 2 2 2
  spline S149 degree 2 poles (9.0674, -216.6953) (8.9452, -216.5989) (8.6413, -216.536) (8.482, -216.536) knots 0 0 0 1 2 2 2
  spline S150 degree 2 poles (8.482, -216.536) (8.2671, -216.536) (7.8633, -216.6656) (7.6669, -216.7879) knots 0 0 0 1 2 2 2
  spline S151 degree 2 poles (7.6669, -216.7879) (7.6632, -216.8546) (7.6558, -216.9806) (7.6558, -217.0769) knots 0 0 0 1 2 2 2
  spline S152 degree 2 poles (7.6558, -217.0769) (7.6558, -217.5511) (7.8411, -218.1328) (7.9818, -218.2847) knots 0 0 0 1 2 2 2
  spline S153 degree 2 poles (7.9818, -218.2847) (8.1115, -218.4292) (8.3931, -218.5441) (8.5524, -218.5441) knots 0 0 0 1 2 2 2
  spline S154 degree 2 poles (8.5524, -218.5441) (8.9229, -218.5441) (9.3786, -218.018) (9.3786, -217.4918) knots 0 0 0 1 2 2 2
  line L127 (12.4427, -214.1721) -> (10.6532, -219.9409)
  line L128 (10.6532, -219.9409) -> (10.1345, -219.9409)
  line L129 (10.1345, -219.9409) -> (11.9166, -214.1721)
  line L130 (11.9166, -214.1721) -> (12.4427, -214.1721)
  line L131 (15.7661, -218.9479) -> (12.9466, -218.9479)
  line L132 (12.9466, -218.9479) -> (12.9466, -218.2995)
  spline S155 degree 2 poles (12.9466, -218.2995) (13.2504, -218.0143) (13.7913, -217.4844) (14.0507, -217.1992) knots 0 0 0 1 2 2 2
  spline S156 degree 2 poles (14.0507, -217.1992) (14.5731, -216.6249) (14.9547, -215.9357) (14.9547, -215.5689) knots 0 0 0 1 2 2 2
  spline S157 degree 2 poles (14.9547, -215.5689) (14.9547, -215.3763) (14.8361, -215.0873) (14.7287, -214.9947) knots 0 0 0 1 2 2 2
  spline S158 degree 2 poles (14.7287, -214.9947) (14.6212, -214.902) (14.3397, -214.8094) (14.1692, -214.8094) knots 0 0 0 1 2 2 2
  spline S159 degree 2 poles (14.1692, -214.8094) (14.0062, -214.8094) (13.6728, -214.8909) (13.5209, -214.9539) knots 0 0 0 1 2 2 2
  spline S160 degree 2 poles (13.5209, -214.9539) (13.3912, -215.0058) (13.1504, -215.154) (13.0763, -215.2058) knots 0 0 0 1 2 2 2
  line L133 (13.0763, -215.2058) -> (13.0429, -215.2058)
  line L134 (13.0429, -215.2058) -> (13.0429, -214.5538)
  spline S161 degree 2 poles (13.0429, -214.5538) (13.2319, -214.4611) (13.9099, -214.2796) (14.2137, -214.2796) knots 0 0 0 1 2 2 2
  spline S162 degree 2 poles (14.2137, -214.2796) (14.8547, -214.2796) (15.5771, -214.9576) (15.5771, -215.5356) knots 0 0 0 1 2 2 2
  spline S163 degree 2 poles (15.5771, -215.5356) (15.5771, -215.8061) (15.4512, -216.2581) (15.34, -216.4507) knots 0 0 0 1 2 2 2
  spline S164 degree 2 poles (15.34, -216.4507) (15.2289, -216.6508) (14.9065, -217.0435) (14.7287, -217.2325) knots 0 0 0 1 2 2 2
  spline S165 degree 2 poles (14.7287, -217.2325) (14.4397, -217.5474) (13.732, -218.2217) (13.5209, -218.4181) knots 0 0 0 1 2 2 2
  line L135 (13.5209, -218.4181) -> (15.7661, -218.4181)
  line L136 (15.7661, -218.4181) -> (15.7661, -218.9479)
  line L137 (19.197, -218.9479) -> (16.3774, -218.9479)
  line L138 (16.3774, -218.9479) -> (16.3774, -218.2995)
  spline S166 degree 2 poles (16.3774, -218.2995) (16.6812, -218.0143) (17.2222, -217.4844) (17.4815, -217.1992) knots 0 0 0 1 2 2 2
  spline S167 degree 2 poles (17.4815, -217.1992) (18.0039, -216.6249) (18.3856, -215.9357) (18.3856, -215.5689) knots 0 0 0 1 2 2 2
  spline S168 degree 2 poles (18.3856, -215.5689) (18.3856, -215.3763) (18.267, -215.0873) (18.1595, -214.9947) knots 0 0 0 1 2 2 2
  spline S169 degree 2 poles (18.1595, -214.9947) (18.0521, -214.902) (17.7705, -214.8094) (17.6001, -214.8094) knots 0 0 0 1 2 2 2
  spline S170 degree 2 poles (17.6001, -214.8094) (17.4371, -214.8094) (17.1036, -214.8909) (16.9517, -214.9539) knots 0 0 0 1 2 2 2
  spline S171 degree 2 poles (16.9517, -214.9539) (16.822, -215.0058) (16.5812, -215.154) (16.5071, -215.2058) knots 0 0 0 1 2 2 2
  line L139 (16.5071, -215.2058) -> (16.4738, -215.2058)
  line L140 (16.4738, -215.2058) -> (16.4738, -214.5538)
  spline S172 degree 2 poles (16.4738, -214.5538) (16.6627, -214.4611) (17.3407, -214.2796) (17.6445, -214.2796) knots 0 0 0 1 2 2 2
  spline S173 degree 2 poles (17.6445, -214.2796) (18.2855, -214.2796) (19.008, -214.9576) (19.008, -215.5356) knots 0 0 0 1 2 2 2
  spline S174 degree 2 poles (19.008, -215.5356) (19.008, -215.8061) (18.882, -216.2581) (18.7709, -216.4507) knots 0 0 0 1 2 2 2
  spline S175 degree 2 poles (18.7709, -216.4507) (18.6597, -216.6508) (18.3374, -217.0435) (18.1595, -217.2325) knots 0 0 0 1 2 2 2
  spline S176 degree 2 poles (18.1595, -217.2325) (17.8706, -217.5474) (17.1629, -218.2217) (16.9517, -218.4181) knots 0 0 0 1 2 2 2